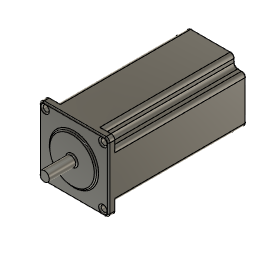
_NEMA23 Stepper (Autodesk Fusion 360 design; units mm, degrees)
Autodesk Fusion 360 part; units mm, degrees
box "BoxPrimitive1" add length 112 width 56.4 height 56 placed x (0, -1, 0) y (1, 0, 0) z (0, 0, 1) at (-31.4, 50, 0)
sketch "Sketch2" plane through (0, -62, 0) normal (0, -1, 0) x (1, 0, 0)
  line L0 (-31.4, 56) -> (-31.4, 0)
  line L1 (-31.4, 0) -> (25, 0)
  line L2 (25, 0) -> (25, 56)
  line L3 (25, 56) -> (-31.4, 56)
  line L4 (-31.4, 0) -> (25, 56) construction
  circle A0 centre (-3.2, 28) radius 19.05
  point P0 (-3.2, 28)
  dimension "d6" = 38.1
  constraint coincident L0.end L1.start
  constraint coincident L2.end L3.start
  constraint midpoint L4 P0
  constraint coincident P0 A0.centre
  measures "d6" diameter of A0
extrude "Extrude1" add sketch "Sketch2" along normal blind 1.6 contours A0
sketch "Sketch3" plane through (0, -63.6, 0) normal (0, -1, 0) x (1, 0, 0)
  circle A0 centre (-3.2, 28) radius 19.05
  circle A1 through (15.85, 28, -1.6) (-12.725, 44.4978, -1.6) (-12.725, 11.5022, -1.6)
  line L0 (-31.4, 56, -1.6) -> (-31.4, 0, -1.6)
  line L1 (-31.4, 0, -1.6) -> (25, 0, -1.6)
  line L2 (25, 0, -1.6) -> (25, 56, -1.6)
  line L3 (25, 56, -1.6) -> (-31.4, 56, -1.6)
  line L4 (25, 56, -113.6) -> (25, 0, -113.6)
  line L5 (25, 0, -113.6) -> (-31.4, 0, -113.6)
  line L6 (-31.4, 0, -113.6) -> (-31.4, 56, -113.6)
  line L7 (-31.4, 56, -113.6) -> (25, 56, -113.6)
  line L8 (-31.4, 0, -1.6) -> (25, 56, -1.6) construction
  circle A2 centre (-3.2, 28) radius 4
  dimension "d9" = 8
  constraint concentric A0 A2
  measures "d9" diameter of A2
extrude "Extrude2" add sketch "Sketch3" along normal blind 22.5 contours A2
sketch "Sketch4" plane through (0, -86.1, 0) normal (0, -1, 0) x (1, 0, 0)
  circle A0 centre (-3.2, 28) radius 4
  line L0 (-7.2, 24) -> (-7.2, 32)
  line L1 (-6.2, 24) -> (-6.2, 32)
  line L2 (-7.2, 32) -> (-6.2, 32)
  line L3 (-7.2, 24) -> (-6.2, 24)
  point P0 (-3.2, 28)
  dimension "d13" = 8
  dimension "d14" = 8
  constraint coincident P0 A0.centre
  constraint perpendicular L1 L2
  constraint perpendicular L1 L3
  measures "d13" distance of L0.start L0.end
  measures "d14" distance of L1.start L1.end
extrude "Extrude3" cut sketch "Sketch4" against normal blind 21 contours A0 L1 | A0 L0 L1 L2 | A0 L0 L1 L3 picked at (-6.4099, 28.5602)
sketch "Sketch5" plane through (0, -62, 0) normal (0, -1, 0) x (1, 0, 0)
  circle A0 centre (-3.2, 28) radius 19.05
  line L0 (-31.4, 56) -> (-31.4, 0)
  line L1 (-31.4, 0) -> (25, 0)
  line L2 (25, 0) -> (25, 56)
  line L3 (25, 56) -> (-31.4, 56)
  line L4 (-22.25, 47.05) -> (-31.4, 47.05)
  line L5 (-31.4, 47.05) -> (-31.4, 56)
  line L6 (-31.4, 56) -> (-22.25, 56)
  line L7 (-22.25, 56) -> (-22.25, 47.05)
  line L8 (15.85, 47.05) -> (25, 47.05)
  line L9 (25, 47.05) -> (25, 56)
  line L10 (25, 56) -> (15.85, 56)
  line L11 (15.85, 56) -> (15.85, 47.05)
  line L12 (15.85, 8.95) -> (25, 8.95)
  line L13 (25, 8.95) -> (25, 0)
  line L14 (25, 0) -> (15.85, 0)
  line L15 (15.85, 0) -> (15.85, 8.95)
  line L16 (-22.25, 8.95) -> (-31.4, 8.95)
  line L17 (-31.4, 8.95) -> (-31.4, 0)
  line L18 (-31.4, 0) -> (-22.25, 0)
  line L19 (-22.25, 0) -> (-22.25, 8.95)
  line L20 (20.35, 51.55) -> (-26.75, 51.55) construction
  line L21 (-26.75, 51.55) -> (-26.75, 4.45) construction
  line L22 (-26.75, 4.45) -> (20.35, 4.45) construction
  line L23 (20.35, 4.45) -> (20.35, 51.55) construction
  line L24 (20.35, 51.55) -> (-26.75, 4.45) construction
  line L25 (-26.75, 51.55) -> (20.35, 4.45) construction
  circle A1 centre (-26.75, 51.55) radius 2.5
  circle A2 centre (20.35, 51.55) radius 2.5
  circle A3 centre (-26.75, 4.45) radius 2.5
  circle A4 centre (20.35, 4.45) radius 2.5
  point P0 (-3.2, 28)
  point P1 (-3.2, 28)
  dimension "d17" = 38.1
  dimension "d18" = 38.1
  dimension "d22" = 47.1
  dimension "d23" = 47.1
  dimension "d24" = 5
  dimension "d25" = 5
  dimension "d26" = 5
  dimension "d27" = 5
  constraint coincident P0 A0.centre
  constraint horizontal L4
  constraint vertical L5
  constraint horizontal L6
  constraint vertical L7
  constraint coincident L0.start L3.end
  constraint horizontal L8
  constraint vertical L9
  constraint horizontal L10
  constraint vertical L11
  constraint coincident L2.end L3.start
  constraint horizontal L12
  constraint vertical L13
  constraint horizontal L14
  constraint vertical L15
  constraint coincident L1.end L2.start
  constraint horizontal L16
  constraint vertical L17
  constraint horizontal L18
  constraint vertical L19
  constraint coincident L0.end L1.start
  constraint perpendicular L20 L21
  constraint parallel L20 L22
  constraint parallel L21 L23
  constraint horizontal L20
  constraint coincident L24 P1
  constraint coincident L25 P1
  constraint coincident P1 P0
  constraint coincident L20.end L21.start
  constraint coincident L20.start L23.end
  constraint coincident L21.end L22.start
  constraint coincident L22.end L23.start
  measures "d17" distance of L4.start L8.start
  measures "d18" distance of L16.start L4.start
  measures "d22" distance of L21.end L22.end
  measures "d23" distance of L20.end L21.end
  measures "d24" diameter of A1
  measures "d25" diameter of A2
  measures "d26" diameter of A3
  measures "d27" diameter of A4
extrude "Extrude4" cut sketch "Sketch5" against normal through all contours L0 L3 L4 L5 L6 L7 | L0 L1 L16 L17 L18 L19 | L2 L3 L8 L9 L10 L11 | L1 L2 L12 L13 L14 L15 | A1 | A2 | A3 | A4
extrude "Extrude5" add sketch "Sketch5" against normal blind 5 contours L0 L3 L4 L5 L6 L7 | L0 L1 L16 L17 L18 L19 | L2 L3 L8 L9 L10 L11 | L1 L2 L12 L13 L14 L15 | A1 | A2 | A3 | A4
extrude "Extrude6" cut sketch "Sketch5" against normal through all contours A1 | A2 | A3 | A4
fillet "Fillet1" radius 3 16 edges at (25, -3.5, 47.05) (25, -59.5, 56) (25, -3.5, 8.95) (15.85, -3.5, 0) (25, -59.5, 0) (-22.25, -3.5, 47.05) (-22.25, -3.5, 56) (-31.4, -3.5, 47.05) (-31.4, -59.5, 0) (-31.4, -3.5, 8.95) (-22.25, -3.5, 0) (15.85, -3.5, 47.05) (-31.4, -59.5, 56) (-22.25, -3.5, 8.95) (15.85, -3.5, 56) (15.85, -3.5, 8.95)
fillet "Fillet2" radius 1 3 faces at (3.3943, 50, 21.5066) (21.95, -62, 28) (10.7475, -63.6, 26.8549)
